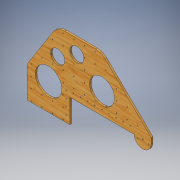
# Autodesk Inventor part: Cote droit Rammasse-Balle
Saved by Autodesk Inventor 2016 (Build 200138000, 138)
## iProperties
Created: 2016-01-24
Part Number: Cote droit Rammasse-Balle
Material: Generic
Document SubType Name: Modeling
Designer: ares-b02
Density: 1 g/cm^3
Appearance: Plywood - New
Author: ares-b02
Autodesk Inventor part; units mm, degrees
ref_plane "YZ Plane" through (0, 0, 0) normal (1, 0, 0) x (0, 1, 0)
ref_plane "XZ Plane" through (0, 0, 0) normal (0, 1, 0) x (-1, 0, 0)
ref_plane "XY Plane" through (0, 0, 0) normal (0, 0, 1) x (1, 0, 0)
sketch "Sketch1" plane through (0, 0, 0) normal (0, 0, 1) x (1, 0, 0)
  line L0 (-426.4123, 367.2389) -> (-151.4123, 97.5421)
  line L1 (-151.4123, 97.5421) -> (-151.4123, 77.5421)
  line L2 (-644.6123, -7.3828) -> (-441.4123, -7.3828)
  line L3 (-441.4123, -7.3828) -> (-441.4123, 77.5421)
  line L4 (-441.4123, 77.5421) -> (-211.4123, 77.5421)
  arc A0 (-211.4123, 77.5421) -> (-151.4123, 77.5421) centre (-181.4123, 77.5421) ccw
  circle A1 centre (-181.4123, 77.5421) radius 2.5
  line L5 (-426.4123, 367.2389) -> (-644.6123, 24.5323)
  line L6 (-644.6123, 24.5323) -> (-644.6123, -7.3828)
  point P0 (0, 0)
  dimension "d0" = 30
  dimension "d1" = 5
  dimension "d2" = 230
  dimension "d3" = 203.2
  dimension "d4" = 84.9249
  dimension "d8" = 20
  dimension "d9" = 290.0849
  dimension "d10" = 245
  dimension "d18" = 31.9151
  constraints: 14 end point, 2 centre point, 2 perpendicular, 2 point on circle, 2 vertical, 1 coincident, 1 tangent
  measures "d0" radius of A0
  measures "d1" diameter of A1
  measures "d2" distance of L3.end L4.end
  measures "d3" distance of L2.start L2.end
  measures "d4" distance of L2.end L3.end
  measures "d8" distance of L0.end L1.end
  measures "d9" distance of L3.end L0.start
  measures "d10" horizontal distance of A0.centre L0.start
  measures "d18" distance of L5.end L2.start
extrude "Extrusion1" add sketch "Sketch1" along normal blind 6.35
sketch "Sketch2" plane through (0, 0, 6.35) normal (0, 0, 1) x (1, 0, 0)
  line L0 (-644.4252, 453.4924) -> (-210.5481, 453.4924)
  line L1 (-210.5481, 453.4924) -> (-210.5481, 272.5421)
  line L2 (-210.5481, 272.5421) -> (-644.4252, 272.5421)
  line L3 (-644.4252, 272.5421) -> (-644.4252, 453.4924)
  circle A0 centre (-181.4123, 77.5421) radius 2.5 projected
  point P0 (0, 0)
  dimension "d11" = 180.9503
  dimension "d12" = 433.8771
  dimension "d13" = 29.1358
  dimension "d14" = 195
  constraints: 8 end point, 2 parallel, 1 horizontal, 1 perpendicular
  measures "d11" distance of L0.end L1.end
  measures "d12" distance of L0.start L0.end
  measures "d13" horizontal distance of A0.centre L1.end
  measures "d14" vertical distance of A0.centre L1.end
extrude "Extrusion2" cut sketch "Sketch2" against normal through all contours L0 L1 L2 L3
fillet "Fillet1" radius 50 1 edges at (-329.8534, 272.5421, 3.175)
fillet "Fillet2" radius 50 1 edges at (-486.7054, 272.5421, 3.175)
hole "Hole4" at (-485.0894, 180.4939, 6.35) direction (0, 0, -1) diameter 50.8 end through all
hole "Hole5" at (-416.3572, 221.7421, 6.35) direction (0, 0, -1) diameter 50.8 end through all
hole "Hole9" at (-517.6123, 88.1466, 6.35) direction (0, 0, -1) diameter 95.25 end through all
hole "Hole10" at (-326.6141, 153.7421, 6.35) direction (0, 0, -1) diameter 88.9 end through all
hole "Hole11" at (-428.7123, 96.5921, 6.35) direction (0, 0, -1) diameter 3.175 end through all
pattern_linear "Rectangular Pattern1" count 9 spacing 25.4 along (1, 0, 0) of "Hole11"
hole "Hole12" at (-454.1123, 15.6423, 6.35) direction (0, 0, -1) diameter 3.175 end through all
pattern_linear "Rectangular Pattern2" count 4 spacing 25.4 along (0, 1, 0) of "Hole12"
sketch "Sketch4" plane through (0, 0, 6.35) normal (0, 0, 1) x (1, 0, 0)
  line L0 (-644.6123, 132.3172) -> (-593.8123, 132.3172)
  line L1 (-593.8123, 132.3172) -> (-593.8123, -7.3828)
  line L2 (-593.8123, -7.3828) -> (-644.6123, -7.3828)
  line L3 (-644.6123, -7.3828) -> (-644.6123, 132.3172)
  line L4 (-644.6123, 24.5323) -> (-644.6123, -7.3828) projected
  line L5 (-644.6123, -7.3828) -> (-441.4123, -7.3828) projected
  point P0 (0, 0)
  dimension "d140" = 0
  dimension "d141" = 0
  dimension "d142" = 139.7
  dimension "d146" = 50.8
  constraints: 8 end point, 2 parallel, 1 horizontal, 1 perpendicular
  measures "d140" distance between parallel lines of L4 L3
  measures "d141" distance between parallel lines of L5 L2
  measures "d142" distance of L2.end L0.start
  measures "d146" distance of L0.start L0.end
extrude "Extrusion3" cut sketch "Sketch4" against normal blind 25.4
fillet "Fillet3" radius 25.4 1 edges at (-593.8123, 104.3192, 3.175)
hole "Hole13" at (-579.2835, -3.4077, 6.35) direction (0, 0, -1) diameter 3.175 end through all
pattern_linear "Rectangular Pattern3" count 12 spacing 38.1 along (1, 0, 0) count 8 spacing 38.1 along (0, 1, 0) of "Hole13"
body "Solid1"
